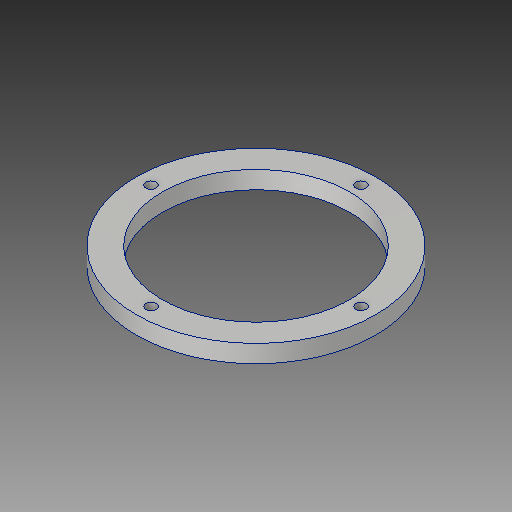
# Autodesk Inventor part: turntable1
Saved by Autodesk Inventor 2019 (Build 230136000, 136)
## iProperties
Created: 2018-11-14
Part Number: turntable1
Material: アルミニウム 6061
Document SubType Name: Modeling
Designer: miyas
Density: 2.7 g/cm^3
Appearance: アルミニウム - フラット
Mass: 90.5751 g
Surface Area: 139.015 cm^2
Volume: 33.5463 cm^3
Author: miyas
Autodesk Inventor part; units mm, degrees
ref_plane "YZ Plane" through (0, 0, 0) normal (1, 0, 0) x (0, 1, 0)
ref_plane "XZ Plane" through (0, 0, 0) normal (0, 1, 0) x (-1, 0, 0)
ref_plane "XY Plane" through (0, 0, 0) normal (0, 0, 1) x (1, 0, 0)
sketch "スケッチ1" plane through (0, 0, 0) normal (0, 1, 0) x (-1, 0, 0)
  circle A0 centre (0, 0) radius 45
  circle A1 centre (0, 0) radius 57.5
  dimension "d0" = 90
  dimension "d1" = 115
  constraints: 2 centre point, 2 coincident
  measures "d0" diameter of A0
  measures "d1" diameter of A1
extrude "押し出し1" add sketch "スケッチ1" along normal blind 8.5
sketch "スケッチ2" plane through (0, 8.5, 0) normal (0, 1, 0) x (1, 0, 0)
  point P0 (0, 0)
  point P1 (-50.5, 0)
  point P2 (0, -50.5)
  point P3 (50.5, 0)
  point P4 (0, 50.5)
  dimension "d4" = 50.5
  dimension "d7" = 360
  constraints: 1 horizontal alignment, 5 other
  measures "d4" distance of point (0, 0) point (-50.5, 0)
hole "穴1" at (-50.5, 8.5, 0) at (0, 8.5, 50.5) at (50.5, 8.5, 0) at (0, 8.5, -50.5) direction (0, -1, 0) diameter 5 end through all
